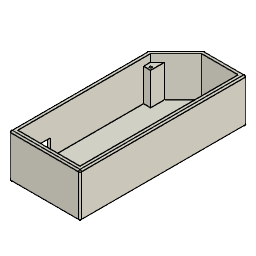
case bottom v25 (Autodesk Fusion 360 design; units mm, degrees)
Autodesk Fusion 360 part; units mm, degrees
box "BoxPrimitive2" add length 118 width 50 height 31.22 placed x (0, 1, 0) y (-1, 0, 0) z (0, 0, 1) at (50, 0, 0)
sketch "Sketch4" plane through (0, 0, 31.22) normal (0, 0, 1) x (-1, 0, 0)
  line L0 (-50, -118) -> (0, -118)
  line L1 (0, -118) -> (0, 0)
  line L2 (0, 0) -> (-50, 0)
  line L3 (-50, 0) -> (-50, -118)
  line L4 (0, -98) -> (-20, -118)
  dimension "d13" = 45
  dimension "d14" = 20
  constraint coincident L1 L4.start
  constraint coincident L0 L4.end
  measures "d13" angle of L1 L4
  measures "d14" distance of L0.end L4.end
extrude "Extrude1" cut sketch "Sketch4" against normal through all contours L0 L1 L4
shell "Shell1" thickness 3 removed faces 1 at (33.3333, 72, 31.22)
fillet "Fillet1" [suppressed]
sketch "Sketch8" plane through (0, 0, 3) normal (0, 0, 1) x (-1, 0, 0)
  line L0 (-21.2426, -115) -> (-3, -96.7574)
  line L1 (-3, -96.7574) -> (-3, -3)
  line L2 (-3, -3) -> (-47, -3)
  line L3 (-47, -3) -> (-47, -115)
  line L4 (-47, -115) -> (-21.2426, -115)
  line L5 (-3, -3) -> (-8, -3)
  line L6 (-8, -3) -> (-8, -8)
  line L7 (-8, -8) -> (-3, -8)
  line L8 (-3, -8) -> (-3, -3)
  line L9 (-47, -3) -> (-42, -3)
  line L10 (-42, -3) -> (-42, -8)
  line L11 (-42, -8) -> (-47, -8)
  line L12 (-47, -8) -> (-47, -3)
  line L13 (-47, -115) -> (-42, -115)
  line L14 (-42, -115) -> (-42, -112)
  line L15 (-42, -112) -> (-47, -112)
  line L16 (-47, -112) -> (-47, -115)
  line L17 (-8, -101.7574) -> (-8, -92)
  line L18 (-8, -92) -> (-3, -92)
  line L19 (-3, -92) -> (-3, -96.7574)
  circle A0 centre (-6, -6) radius 0.8
  circle A1 centre (-44, -6) radius 0.8
  circle A2 centre (-6, -94) radius 0.8
  circle A3 centre (-44, -114) radius 0.8
  line L20 (-6, -94) -> (-6, -6) construction
  line L21 (-6, -6) -> (-44, -6) construction
  line L22 (-44, -6) -> (-44, -114) construction
  line L23 (-3, -96.7574) -> (-8, -101.7574)
  dimension "d20" = 1.6
  dimension "d21" = 1.6
  dimension "d22" = 1.6
  dimension "d23" = 1.6
  dimension "d24" = 88
  dimension "d25" = 108
  dimension "d26" = 38
  dimension "d27" = 3
  dimension "d28" = 3
  dimension "d29" = 2
  dimension "d30" = 2
  dimension "d31" = 2
  dimension "d32" = 2
  dimension "d33" = 2
  dimension "d34" = 2
  dimension "d35" = 2
  dimension "d36" = 2
  constraint horizontal L5
  constraint vertical L6
  constraint horizontal L7
  constraint vertical L8
  constraint coincident L1.end L2.start
  constraint horizontal L9
  constraint vertical L10
  constraint horizontal L11
  constraint vertical L12
  constraint coincident L2.end L3.start
  constraint horizontal L13
  constraint vertical L14
  constraint horizontal L15
  constraint vertical L16
  constraint coincident L3.end L4.start
  constraint vertical L17
  constraint horizontal L18
  constraint vertical L19
  constraint coincident L0.end L1.start
  constraint coincident A2.centre L20.start
  constraint coincident A0.centre L20.end
  constraint coincident A1.centre L21.end
  constraint coincident A3.centre L22.end
  constraint perpendicular L11 L22
  constraint perpendicular L20 L21
  constraint perpendicular L21 L22
  constraint coincident L0 L17.start
  measures "d20" diameter of A2
  measures "d21" diameter of A0
  measures "d22" diameter of A1
  measures "d23" diameter of A3
  measures "d24" vertical distance of A2.centre A0.centre
  measures "d25" distance of A1.centre A3.centre
  measures "d26" distance of A0.centre A1.centre
  measures "d27" distance of L5 A0.centre
  measures "d28" distance of L8 A0.centre
  measures "d29" distance of L17 A2.centre
  measures "d30" distance of L18 A2.centre
  measures "d31" distance of L7 A0.centre
  measures "d32" distance of L6 A0.centre
  measures "d33" distance of L10 A1.centre
  measures "d34" distance of L11 A1.centre
  measures "d35" distance of L15 A3.centre
  measures "d36" distance of L14 A3.centre
extrude "Extrude2" add sketch "Sketch8" along normal blind 22.97 contours L0 L1 L17 L18 L19 L23 | L3 L4 L13 L14 L15 L16 | L1 L2 L5 L6 L7 L8 | L2 L3 L9 L10 L11 L12
sketch "Sketch9" plane through (0, 0, 0) normal (0, 0, -1) x (1, 0, 0)
  line L0 (0, -98) -> (20, -118)
  line L1 (20, -118) -> (50, -118)
  line L2 (50, -118) -> (50, 0)
  line L3 (50, 0) -> (0, 0)
  line L4 (0, 0) -> (0, -98)
  line L5 (28.3325, -7.8768) -> (16.6957, -5.9578)
  line L6 (22.7114, -11.9325) -> (26.2566, -10.6775)
  line L7 (26.2566, -10.6775) -> (27.4392, -11.1538)
  line L8 (27.4392, -11.1538) -> (36.9885, -11.5516)
  arc A0 (38.3483, -13.5661) -> (20.454, -14.0111) centre (30.2312, -47.1733) ccw
  arc A1 (37.5209, -12.1447) -> (20.454, -13.3831) centre (31.9438, -53.5051) ccw
  line L9 (31.8615, -15.1353) -> (26.0225, -17.969)
  line L10 (31.9317, -14.3791) -> (25.7086, -17.3991)
  line L11 (34.4849, -15.383) -> (30.2593, -18.4958)
  line L12 (29.5231, -19.504) -> (29.9701, -19.36)
  line L13 (30.2593, -18.4958) -> (31.3861, -16.3549)
  line L14 (29.9701, -19.36) -> (35.0187, -15.6247)
  arc A2 (38.3483, -13.5661) -> (27.9396, -32.1129) centre (59.5863, -37.6793) ccw
  line L15 (31.1446, -16.1148) -> (27.0953, -20.6786)
  line L16 (31.9686, -15.3663) -> (31.8615, -15.1353)
  line L17 (31.9686, -15.3663) -> (31.1446, -16.1148)
  line L18 (31.3861, -16.3549) -> (33.4826, -15.383)
  line L19 (32.4076, -15.2488) -> (31.9317, -14.3791)
  line L20 (36.9885, -11.5516) -> (28.3325, -7.8768)
  line L21 (33.4826, -15.383) -> (34.4849, -15.383)
  line L22 (34.5696, -14.7695) -> (33.1791, -14.9172)
  line L23 (33.1791, -14.9172) -> (32.4076, -15.2488)
  line L24 (35.0187, -15.6247) -> (34.5696, -14.7695)
  arc A3 (38.3483, -13.5661) -> (36.9885, -11.5516) centre (32.8104, -15.8378) ccw
  line L25 (28.1132, -29.1272) -> (28.1132, -23.3533)
  line L26 (27.5328, -28.9241) -> (27.5328, -23.6176)
  line L27 (27.085, -29.5331) -> (27.5328, -28.9241)
  line L28 (27.4109, -30.0917) -> (28.1132, -29.1272)
  line L29 (24.5784, -29.9341) -> (27.085, -29.5331)
  line L30 (24.5158, -30.5607) -> (27.4109, -30.0917)
  line L31 (23.6387, -30.2407) -> (23.6387, -27.7298)
  line L32 (23.1458, -30.514) -> (23.1983, -27.6294)
  line L33 (24.1967, -29.9228) -> (23.6387, -30.2407)
  line L34 (22.5456, -31.4617) -> (24.5158, -30.5607)
  line L35 (12.6028, -35.9118) -> (23.1458, -30.514)
  line L36 (21.4481, -33.0831) -> (21.9433, -31.6978)
  line L37 (21.9223, -33.3247) -> (22.5456, -31.4617)
  line L38 (21.9433, -31.6978) -> (17.0979, -34.522)
  line L39 (23.1983, -27.6294) -> (17.7482, -27.7629)
  line L40 (17.7482, -27.7629) -> (17.897, -29.4332)
  line L41 (10.7404, -27.692) -> (17.202, -27.8268)
  line L42 (17.202, -27.8268) -> (15.7726, -29.1413)
  line L43 (17.897, -29.4332) -> (13.5732, -31.748)
  line L44 (17.9222, -24.9733) -> (15.4702, -27.1378)
  line L45 (16.2376, -27.2652) -> (18.3901, -25.3238)
  line L46 (17.8576, -27.2652) -> (16.2376, -27.2652)
  line L47 (15.4702, -27.1378) -> (10.651, -27.1378)
  line L48 (21.0824, -25.768) -> (17.8576, -27.2652)
  line L49 (18.699, -24.6635) -> (17.9222, -24.9733)
  line L50 (19.5563, -25.3508) -> (18.3901, -25.3238)
  line L51 (21.625, -25.2319) -> (18.699, -24.6635)
  line L52 (15.8531, -37.6407) -> (21.4481, -33.0831)
  line L53 (14.9681, -39.0787) -> (21.9223, -33.3247)
  arc A4 (23.2732, -38.2883) -> (7.4661, -42.8136) centre (38.8428, -122.5446) ccw
  line L54 (17.0979, -34.522) -> (16.161, -35.633)
  line L55 (16.1508, -34.7578) -> (15.6602, -35.5146)
  line L56 (12.347, -36.5769) -> (16.1508, -34.7578)
  line L57 (11.4445, -31.3677) -> (13.2435, -30.3149)
  line L58 (13.2435, -30.3149) -> (12.0508, -30.0117)
  line L59 (15.4081, -30.1329) -> (11.1823, -28.6544)
  line L60 (15.7726, -29.1413) -> (15.4081, -30.1329)
  line L61 (14.344, -30.4027) -> (14.5718, -30.4895)
  line L62 (14.5718, -30.4895) -> (12.2276, -31.9937)
  line L63 (11.6559, -31.8757) -> (14.344, -30.4027)
  arc A5 (12.6435, -18.9881) -> (10.0006, -24.5429) centre (47.732, -39.0883) ccw
  line L64 (7.4417, -19.2636) -> (11.0189, -17.8439)
  line L65 (10.1316, -16.4242) -> (7.4417, -19.2636)
  line L66 (11.6195, -29.5535) -> (9.1936, -30.2004)
  line L67 (11.1411, -29.257) -> (11.6195, -29.5535)
  line L68 (12.0508, -30.0117) -> (9.5939, -30.6948)
  line L69 (12.2484, -35.4996) -> (12.6028, -35.9118)
  line L70 (9.2522, -35.7499) -> (13.288, -34.6055)
  line L71 (13.288, -34.6055) -> (12.2484, -35.4996)
  line L72 (11.6135, -35.6017) -> (12.347, -36.5769)
  line L73 (9.0139, -36.3389) -> (11.6135, -35.6017)
  line L74 (12.2276, -31.9937) -> (7.8364, -35.5922)
  line L75 (13.5732, -31.748) -> (8.8527, -35.4113)
  line L76 (8.7976, -31.4911) -> (11.4445, -31.3677)
  line L77 (7.9005, -32.1114) -> (11.6559, -31.8757)
  line L78 (10.651, -27.1378) -> (8.7642, -28.2839)
  line L79 (8.6125, -28.8467) -> (11.1411, -29.257)
  line L80 (11.1823, -28.6544) -> (9.535, -28.4598)
  line L81 (9.535, -28.4598) -> (10.7404, -27.692)
  line L82 (19.55, -27.3726) -> (24.1014, -24.47)
  line L83 (23.3473, -27.2795) -> (19.55, -27.3726)
  line L84 (21.0824, -25.768) -> (19.5563, -25.3508)
  arc A6 (27.4538, -37.6221) -> (23.8479, -38.1842) centre (38.8428, -122.5446) ccw
  line L85 (23.6034, -37.4403) -> (23.2732, -38.2883)
  line L86 (23.8479, -38.1842) -> (23.6034, -37.4403)
  line L87 (23.6387, -27.7298) -> (24.1902, -27.2626)
  line L88 (25.8044, -23.9941) -> (23.3473, -27.2795)
  line L89 (24.1902, -27.2626) -> (24.1967, -29.9228)
  line L90 (24.498, -26.8264) -> (24.5784, -29.9341)
  line L91 (26.2543, -23.9514) -> (24.498, -26.8264)
  line L92 (22.8119, -24.7074) -> (25.5541, -23.5562)
  line L93 (24.1014, -24.47) -> (25.8044, -23.9941)
  line L94 (26.9576, -33.396) -> (27.8165, -32.865)
  line L95 (27.7405, -33.396) -> (26.9576, -33.396)
  arc A7 (27.7405, -33.396) -> (27.4538, -37.6221) centre (59.5863, -37.6793) ccw
  line L96 (22.1357, -24.984) -> (21.625, -25.2319)
  line L97 (24.4245, -19.9256) -> (22.8119, -24.7074)
  line L98 (23.8544, -19.7907) -> (22.1357, -24.984)
  arc A8 (20.454, -14.0111) -> (17.6701, -18.9239) centre (22.3808, -18.348) ccw
  arc A9 (27.878, -32.4751) -> (27.8165, -32.865) centre (59.5863, -37.6793) ccw
  line L99 (27.5328, -32.3644) -> (27.9396, -32.1129)
  line L100 (27.878, -32.4751) -> (27.5328, -32.3644)
  line L101 (25.5541, -23.5562) -> (25.406, -18.762)
  line L102 (25.7086, -17.3991) -> (23.8544, -19.7907)
  line L103 (26.0225, -17.969) -> (26.0225, -23.0262)
  line L104 (25.406, -18.762) -> (24.4245, -19.9256)
  line L105 (28.1132, -23.3533) -> (29.5231, -19.504)
  line L106 (27.5328, -23.6176) -> (26.2543, -23.9514)
  line L107 (27.0273, -23.2889) -> (27.0953, -20.6786)
  line L108 (28.8463, -19.5223) -> (27.4069, -22.9365)
  line L109 (26.0225, -23.0262) -> (26.7772, -23.4268)
  line L110 (26.7772, -23.4268) -> (27.0273, -23.2889)
  line L111 (27.4069, -22.9365) -> (27.4069, -20.8574)
  arc A10 (20.454, -13.3831) -> (12.6435, -18.9881) centre (24.3939, -27.1179) ccw
  line L112 (19.7172, -12.6227) -> (19.7172, -11.8737)
  line L113 (15.0258, -14.8817) -> (19.7172, -12.6227)
  line L114 (18.7863, -12.2032) -> (20.3157, -11.6618)
  line L115 (11.0189, -17.8439) -> (13.8252, -14.8817)
  line L116 (15.6602, -35.5146) -> (14.9681, -39.0787)
  line L117 (16.161, -35.633) -> (15.8531, -37.6407)
  line L118 (8.8527, -35.4113) -> (9.2522, -35.7499)
  line L119 (7.8364, -35.5922) -> (9.0139, -36.3389)
  arc A11 (9.754, -25.1995) -> (7.4661, -42.8136) centre (47.732, -39.0883) ccw
  line L120 (8.3648, -31.2718) -> (8.0567, -31.2718)
  line L121 (9.1936, -30.2004) -> (8.3648, -31.2718)
  line L122 (9.5939, -30.6948) -> (8.7976, -31.4911)
  line L123 (10.4024, -24.9575) -> (10.0006, -24.5429)
  line L124 (9.754, -25.1995) -> (10.4024, -24.9575)
  line L125 (9.4778, -15.1166) -> (12.56, -15.1166)
  line L126 (14.8203, -12.875) -> (9.4778, -15.1166)
  line L127 (13.0733, -8.9018) -> (7.8062, -11.366)
  line L128 (7.8062, -11.366) -> (16.5254, -11.366)
  line L129 (9.8891, -12.8192) -> (11.83, -11.366)
  line L130 (13.1346, -12.4801) -> (9.8891, -12.8192)
  line L131 (12.56, -15.1166) -> (10.1316, -16.4242)
  line L132 (7.3456, -6.9173) -> (14.7331, -9.4768)
  line L133 (17.3082, -8.0197) -> (7.3456, -6.9173)
  line L134 (13.2566, -11.366) -> (16.041, -10.2034)
  line L135 (16.5254, -11.366) -> (13.1346, -12.4801)
  line L136 (12.1466, -12.5833) -> (14.8203, -12.875)
  line L137 (16.6957, -5.9578) -> (25.2702, -10.0817)
  line L138 (21.5546, -9.7142) -> (17.3082, -8.0197)
  line L139 (16.041, -10.2034) -> (18.9958, -10.2034)
  line L140 (20.3157, -11.6618) -> (22.7114, -11.9325)
  line L141 (25.2702, -10.0817) -> (21.5546, -9.7142)
  line L142 (27.4069, -20.8574) -> (28.8463, -19.5223)
  line L143 (13.8252, -14.8817) -> (15.0258, -14.8817)
  arc A12 (17.6701, -18.9239) -> (12.8306, -18.724) centre (15.073, -23.12) ccw
  constraint horizontal L143
  constraint coincident L78.end A11
  constraint coincident L79.start A11
  constraint coincident L120.end A11
  constraint horizontal L120
  constraint coincident L77.start A11
  constraint coincident A1.start A3
  constraint coincident A10 A12.end
  constraint coincident L112.end L114
  constraint vertical L112
  constraint coincident L136.start L130
  constraint coincident L129.end L128
  constraint coincident L134.start L128
  constraint coincident L127.start L132
sketch "Sketch10" plane through (0, 0, 0) normal (0, 0, -1) x (1, 0, 0)
  arc A0 (29.3353, -78.0058) -> (15.7918, -77.9796) centre (22.5831, -67.9014) ccw
  arc A1 (29.3353, -78.0058) -> (15.7918, -77.9796) centre (22.5878, -65.4216) ccw
  arc A2 (27.0601, -65.4463) -> (27.7519, -64.3503) centre (26.7899, -64.5093) ccw
  arc A3 (27.7519, -64.3503) -> (27.3786, -62.2005) centre (-105.7135, -86.4189) ccw
  arc A4 (27.3786, -62.2005) -> (25.0705, -56.7871) centre (10.293, -66.2867) ccw
  arc A5 (25.0705, -56.7871) -> (21.0429, -56.6052) centre (22.6241, -66.2744) ccw
  arc A6 (21.0429, -56.6052) -> (22.6922, -63.2187) centre (25.8712, -58.9135) ccw
  arc A7 (22.6922, -63.2187) -> (21.1458, -63.9951) centre (22.795, -65.3517) ccw
  arc A8 (21.1458, -63.9951) -> (19.7225, -62.833) centre (19.3059, -64.796) ccw
  arc A9 (19.7225, -62.833) -> (20.5193, -61.4176) centre (18.6029, -61.2708) ccw
  arc A10 (20.5193, -61.4176) -> (20.1091, -59.572) centre (17.2791, -61.1694) ccw
  arc A11 (20.1091, -59.572) -> (19.6772, -59.3951) centre (19.7913, -59.7322) ccw
  arc A12 (19.6772, -59.3951) -> (17.3368, -63.1383) centre (25.6865, -65.7555) ccw
  arc A13 (17.3368, -63.1383) -> (17.951, -64.1792) centre (19.1567, -62.7662) ccw
  arc A14 (18.0097, -64.1792) -> (17.951, -65.5132) centre (18.9263, -64.8878) ccw
  arc A15 (17.951, -65.5132) -> (18.0682, -67.483) centre (19.5154, -66.4085) ccw
  arc A16 (18.0682, -67.483) -> (17.0695, -70.1228) centre (19.6604, -69.5943) ccw
  arc A17 (17.0695, -70.1228) -> (19.1934, -69.7688) centre (17.7756, -67.8111) ccw
  arc A18 (19.1934, -69.7688) -> (20.0624, -70.2249) centre (19.8782, -69.52) ccw
  line L0 (20.0624, -70.2249) -> (22.2108, -69.6637)
  arc A19 (22.2108, -69.6637) -> (21.2107, -78.7003) centre (42.8658, -76.5232) ccw
  arc A20 (21.2107, -78.7003) -> (24.0016, -84.3282) centre (30.4857, -77.6068) ccw
  arc A21 (23.8271, -82.4068) -> (24.0016, -84.3282) centre (31.4292, -82.6849) ccw
  arc A22 (22.2969, -76.4593) -> (23.8271, -82.4068) centre (31.0143, -77.3871) ccw
  line L1 (22.2969, -76.4593) -> (22.8093, -71.6449)
  arc A23 (22.2969, -76.4593) -> (23.769, -81.2842) centre (28.7046, -77.1413) ccw
  arc A24 (25.5069, -68.5131) -> (23.769, -81.2842) centre (124.9555, -88.5499) ccw
  arc A25 (25.5069, -68.5131) -> (26.4147, -67.1738) centre (25.2816, -67.3831) ccw
  arc A26 (26.4147, -67.1738) -> (27.0601, -65.4463) centre (25.1598, -65.7207) ccw
  arc A27 (21.471, -66.7888) -> (27.0601, -65.4463) centre (9.3716, -4.1096) ccw
  arc A28 (19.5409, -66.1805) -> (21.471, -66.7888) centre (21.0633, -64.7162) ccw
  arc A29 (18.2746, -64.7162) -> (19.5409, -66.1805) centre (32.7319, -53.4929) ccw
  arc A30 (18.2746, -64.7162) -> (20.0475, -68.09) centre (27.4635, -62.0404) ccw
  arc A31 (20.0475, -68.09) -> (25.8988, -66.8412) centre (18.7594, -47.7231) ccw
  arc A32 (25.8988, -66.8412) -> (26.7171, -65.5442) centre (25.6274, -65.7632) ccw
  arc A33 (18.3317, -68.0195) -> (18.946, -69.352) centre (24.9328, -65.784) ccw
  arc A34 (18.3317, -68.0195) -> (17.5617, -69.7759) centre (19.2681, -69.4771) ccw
  arc A35 (17.5617, -69.7759) -> (18.946, -69.352) centre (17.5376, -67.2251) ccw
  arc A36 (20.6603, -76.6665) -> (21.0876, -81.2244) centre (29.3864, -78.1474) ccw
  arc A37 (18.684, -76.079) -> (20.6603, -76.6665) centre (21.645, -69.7369) ccw
  arc A38 (18.684, -76.079) -> (21.0876, -81.2244) centre (21.8708, -77.7245) ccw
  arc A39 (21.0876, -82.1859) -> (17.9923, -81.1673) centre (18.846, -83.7855) ccw
  arc A40 (17.9923, -81.1673) -> (15.5551, -83.4747) centre (23.5806, -89.5109) ccw
  arc A41 (15.5551, -83.4747) -> (21.2372, -83.1863) centre (18.3234, -81.8973) ccw
  arc A42 (19.191, -82.9109) -> (21.2372, -83.1863) centre (20.5169, -80.7989) ccw
  arc A43 (21.0876, -82.1859) -> (19.191, -82.9109) centre (20.7818, -84.229) ccw
  arc A44 (22.1829, -83.3782) -> (21.561, -87.2187) centre (23.3897, -85.5442) ccw
  arc A45 (23.2018, -89.037) -> (21.561, -87.2187) centre (-102.4758, -200.7978) ccw
  arc A46 (23.2018, -89.037) -> (24.8742, -86.4323) centre (19.6123, -84.8932) ccw
  arc A47 (24.8742, -86.4323) -> (23.2019, -84.764) centre (-104.4181, -214.3653) ccw
  arc A48 (22.3848, -84.7071) -> (23.2019, -84.764) centre (22.7901, -84.7823) ccw
  arc A49 (22.3848, -84.7071) -> (22.1829, -83.3782) centre (20.3707, -84.3332) ccw
  arc A50 (24.5343, -82.8394) -> (27.7931, -84.8906) centre (26.7045, -83.0059) ccw
  arc A51 (29.5909, -84.4193) -> (27.7931, -84.8906) centre (29.5521, -87.9359) ccw
  arc A52 (29.5909, -84.4193) -> (24.6094, -81.5737) centre (26.2351, -84.5109) ccw
  arc A53 (26.2684, -82.8592) -> (24.6094, -81.5737) centre (23.2245, -85.0742) ccw
  arc A54 (24.5343, -82.8394) -> (26.2684, -82.8592) centre (25.4174, -81.4481) ccw
  arc A55 (24.6094, -80.9033) -> (27.2353, -78.0586) centre (24.6682, -78.3232) ccw
  arc A56 (27.1971, -75.5191) -> (27.2353, -78.0586) centre (41.6634, -76.5714) ccw
  arc A57 (27.1971, -75.5191) -> (25.0194, -78.1016) centre (27.1969, -77.7283) ccw
  arc A58 (24.9069, -79.0983) -> (25.0194, -78.1016) centre (23.2447, -78.4059) ccw
  arc A59 (24.9069, -79.0983) -> (25.1055, -79.3156) centre (26.9196, -77.4584) ccw
  arc A60 (25.1055, -79.3156) -> (24.6094, -80.9033) centre (27.7204, -81.004) ccw
  constraint tangent A2 A3
  constraint tangent A2 A4
  constraint tangent A9 A10
  constraint tangent A13 A15
  constraint tangent A18 L0
  constraint tangent A20 A22
  constraint tangent A22 L1
  constraint tangent L1 A23
  constraint tangent A2 A27
  constraint tangent A28 A29
  constraint coincident A27 A32.end
  constraint tangent A44 A45
  constraint tangent A45 A47
  constraint tangent A48 A49
  constraint tangent A50 A51
  constraint tangent A55 A56
  constraint tangent A57 A58
  constraint tangent A57 A59
sketch "Sketch12" plane through (0, 0, 0) normal (-1, 0, 0) x (0, -1, 0)
  line L0 (-98, 31.22) -> (-98, 0)
  line L1 (-98, 0) -> (0, 0)
  line L2 (0, 0) -> (0, 31.22)
  line L3 (0, 31.22) -> (-98, 31.22)
  line L4 (-26, 15) -> (-8, 15)
  line L5 (-8, 15) -> (-8, 3)
  line L6 (-8, 3) -> (-26, 3)
  line L7 (-26, 3) -> (-26, 15)
  dimension "d43" = 18
  dimension "d44" = 12
  dimension "d45" = 8
  dimension "d46" = 3
  constraint horizontal L4
  constraint vertical L5
  constraint horizontal L6
  constraint vertical L7
  measures "d43" distance of L5.end L6.end
  measures "d44" distance of L4.end L5.end
  measures "d45" distance of L2 L5
  measures "d46" distance of L1 L6
thread "Thread1" "ISO Metric profile 2.0 M2x0.4 M2x0.4 6H" major diameter 2.074 minor diameter 1.623 pitch 0.4 angle 60 resizes the face on face at (5.204, 6.0797, 10.6567) on face at (43.9801, 5.2002, 18.3133) on face at (43.2974, 113.6174, 18.3133) on face at (5.2974, 93.6174, 18.3133)
extrude "Extrude3" cut sketch "Sketch12" against normal blind 3 contours L4 L5 L6 L7
fillet "Fillet2" radius 1 6 faces at (50, 78.6667, 10.4067) (33.3333, 0, 10.4067) (33.3333, 72, 0) (30, 118, 20.8133) (6.6667, 104.6667, 20.8133) (0, 74, 15.4067)
